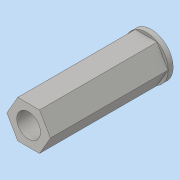
# Autodesk Inventor part: BrushlessMotor_HexHub
Saved by Autodesk Inventor 2016 (Build 200138000, 138)
## iProperties
Created: 2016-08-08
Part Number: BrushlessMotor_HexHub
Material: Generic
Document SubType Name: Modeling
Designer: rahuliyer
Density: 1 g/cm^3
Appearance: Default
Author: rahuliyer
Autodesk Inventor part; units mm, degrees
ref_plane "YZ Plane" through (0, 0, 0) normal (1, 0, 0) x (0, 1, 0)
ref_plane "XZ Plane" through (0, 0, 0) normal (0, 1, 0) x (-1, 0, 0)
ref_plane "XY Plane" through (0, 0, 0) normal (0, 0, 1) x (1, 0, 0)
sketch "Sketch2" plane through (0, 0, 0) normal (0, 0, 1) x (1, 0, 0)
  line L0 (2.7496, 4.7625) -> (5.4993, 0)
  line L1 (5.4993, 0) -> (2.7496, -4.7625)
  line L2 (2.7496, -4.7625) -> (-2.7496, -4.7625)
  line L3 (-2.7496, -4.7625) -> (-5.4993, 0)
  line L4 (-5.4993, 0) -> (-2.7496, 4.7625)
  line L5 (-2.7496, 4.7625) -> (2.7496, 4.7625)
  circle A0 centre (0, 0) radius 3
  line L6 (-7.699, 0) -> (7.699, 0) projected
  line L7 (0, -6.6675) -> (0, 6.6675) projected
  point P0 (0, 3)
  dimension "d0" = 6
  dimension "d1" = 9.525
  constraints: 12 end point, 2 coincident, 1 horizontal, 1 point on line, 1 vertical alignment, 15 other
  measures "d1" distance between parallel lines of L5 L2
extrude "Extrusion1" add sketch "Sketch2" along normal mid plane 31 contours L0 L6 A0 L7 L5 | L1 L2 L7 A0 L6 | L7 A0 L6 L4 L5 | L2 L3 L6 A0 L7
sketch "Sketch3" plane through (0, 0, -15.5) normal (0, 0, -1) x (-1, 0, 0)
  circle A0 centre (0, 0) radius 5.4993
  circle A1 centre (0, 0) radius 3 projected
  line L0 (-2.7496, 4.7625) -> (-5.4993, 0) projected
  line L1 (-5.4993, 0) -> (-2.7496, -4.7625) projected
  line L2 (-2.7496, -4.7625) -> (2.7496, -4.7625) projected
  line L3 (2.7496, -4.7625) -> (5.4993, 0) projected
  line L4 (5.4993, 0) -> (2.7496, 4.7625) projected
  line L5 (2.7496, 4.7625) -> (-2.7496, 4.7625) projected
  constraints: 1 coincident, 1 horizontal alignment, 2 other
extrude "Extrusion2" add sketch "Sketch3" against normal blind 1.27 contours L4 A0 | A0 L3 | L5 A0 | A0 L2 | L0 A0 | A0 L1
body "Solid1"
